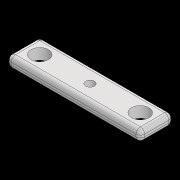
# Autodesk Inventor part: Steering_BottomPlate
Saved by Autodesk Inventor 2022 (Build 260153000, 153)
## iProperties
Created: 2022-07-22
Part Number: Steering_BottomPlate
Material: Generic
Document SubType Name: Modeling
Designer: tandu
Density: 1 g/cm^3
Appearance: Default
Author: tandu
Autodesk Inventor part; units mm, degrees
ref_plane "YZ Plane" through (0, 0, 0) normal (1, 0, 0) x (0, 1, 0)
ref_plane "XZ Plane" through (0, 0, 0) normal (0, 1, 0) x (-1, 0, 0)
ref_plane "XY Plane" through (0, 0, 0) normal (0, 0, 1) x (1, 0, 0)
sketch "Sketch1" plane through (0, 0, 0) normal (0, 1, 0) x (-1, 0, 0)
  line L0 (7.747, 1.905) -> (-7.747, 1.905)
  line L1 (-7.747, 1.905) -> (-7.747, -1.905)
  line L2 (-7.747, -1.905) -> (7.747, -1.905)
  line L3 (7.747, -1.905) -> (7.747, 1.905)
  line L4 (7.747, 1.905) -> (-7.747, -1.905) construction
  line L5 (-7.747, 1.905) -> (7.747, -1.905) construction
  circle A0 centre (0, 0) radius 0.508
  circle A1 centre (-5.842, 0) radius 1.016
  line L6 (-3.937, 1.905) -> (-7.747, 1.905)
  line L7 (-7.747, 1.905) -> (-7.747, -1.905)
  line L8 (-7.747, -1.905) -> (-3.937, -1.905)
  line L9 (-3.937, -1.905) -> (-3.937, 1.905) construction
  line L10 (-3.937, 1.905) -> (-7.747, -1.905) construction
  line L11 (-7.747, 1.905) -> (-3.937, -1.905) construction
  line L12 (0, -1.905) -> (0, 1.905) construction
  circle A2 centre (5.842, 0) radius 1.016
  point P0 (0, 0)
  dimension "d0" = 15.494
  dimension "d1" = 3.81
  dimension "d2" = 1.016
  dimension "d3" = 2.032
  constraints: 26 end point, 7 midpoint, 4 parallel, 3 centre point, 3 perpendicular, 2 horizontal, 1 coincident, 1 horizontal alignment, 1 symmetric about line, 1 other
  measures "d0" distance of L2.end L1.end
  measures "d1" distance of L1.end L0.end
  measures "d2" diameter of A0
  measures "d3" diameter of A1
extrude "Extrusion1" add sketch "Sketch1" along normal blind 1.27
fillet "Fillet1" radius 0.5 12 edges at (-7.747, 0.635, 1.905) (-7.747, 0.635, -1.905) (7.747, 0.635, 1.905) (7.747, 0.635, -1.905) (0, 0, 1.905) (-7.747, 0, 0) (0, 0, -1.905) (7.747, 0, 0) (0, 1.27, 1.905) (7.747, 1.27, 0) (0, 1.27, -1.905) (-7.747, 1.27, 0)
body "Solid1"
